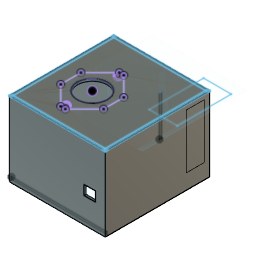
spws box v4 (Autodesk Fusion 360 design; units mm, degrees)
Autodesk Fusion 360 part; units mm, degrees
note: some values were not read from the file. Set by a fixed rule: which sketch regions a step uses.
cylinder "CylinderPrimitive1" add diameter 27.8 height 37 placed x (1, 0, 0) y (0, 1, 0) z (0, 0, 1) at (49.5584, -15.2977, 0) makes body 1
sketch "Sketch2" plane through (0, 0, 0) normal (0, 0, -1) x (1, 0, 0)
  circle A0 centre (49.5584, 15.2977) radius 13.9
  line L0 (38.0977, 16.5) -> (39.0977, 16.5)
  line L1 (39.0977, 16.5) -> (39.0977, 13.5)
  line L2 (39.0977, 13.5) -> (38.0977, 13.5)
  line L3 (38.0977, 13.5) -> (38.0977, 16.5)
  line L4 (60.0977, 16.5) -> (61.0977, 16.5)
  line L5 (61.0977, 16.5) -> (61.0977, 13.5)
  line L6 (61.0977, 13.5) -> (60.0977, 13.5)
  line L7 (60.0977, 13.5) -> (60.0977, 16.5)
  line L8 (35.6613, 15.0104) -> (63.4554, 15.0104) construction
  dimension "d4" = 1
  dimension "d5" = 3
  dimension "d6" = 1
  dimension "d7" = 3
  dimension "d8" = 23
  constraint horizontal L0
  constraint vertical L1
  constraint horizontal L2
  constraint vertical L3
  constraint horizontal L4
  constraint vertical L5
  constraint horizontal L6
  constraint vertical L7
  constraint coincident A0 L8.start
  constraint coincident A0 L8.end
  constraint perpendicular L3 L8
  constraint collinear L0 L4
  measures "d4" distance of L0.start L0.end
  measures "d5" distance of L0.start L2.end
  measures "d6" distance of L4.start L4.end
  measures "d7" distance of L4.start L6.end
  measures "d8" distance of L3 L5
extrude "Extrude1" add sketch "Sketch2" along normal blind 9 contours L0 L1 L2 L3 | L4 L5 L6 L7 bodies 1
sketch "Sketch3" plane through (0, 0, 37) normal (0, 0, 1) x (-1, 0, 0)
  circle A0 centre (-49.5584, 15.2977) radius 13.9
  line L0 (-29.4469, 24.7508) -> (-29.4469, 5.8367)
  line L1 (-29.4469, 5.8367) -> (-47.4256, -12.142)
  line L2 (-51.6682, -12.142) -> (-69.6469, 5.8367)
  line L3 (-69.6469, 5.8367) -> (-69.6469, 24.7508)
  line L4 (-69.6469, 24.7508) -> (-51.6682, 42.7295)
  line L5 (-47.4256, 42.7295) -> (-29.4469, 24.7508)
  line L6 (-49.5469, -14.2633) -> (-49.5469, 44.8508) construction
  line L7 (-29.4469, 15.2937) -> (-69.6469, 15.2937) construction
  arc A1 (-51.6682, -12.142) -> (-47.4256, -12.142) centre (-49.5469, -10.0207) ccw
  arc A2 (-47.4256, 42.7295) -> (-51.6682, 42.7295) centre (-49.5469, 40.6081) ccw
  circle A3 centre (-49.5584, 15.2977) radius 1.15
  circle A4 centre (-49.5469, 39.4977) radius 1.4
  circle A5 centre (-49.5469, -8.9023) radius 1.4
  dimension "d11" = 40.2
  dimension "d14" = 41.8
  dimension "d15" = 41.8
  dimension "d19" = 3
  dimension "d22" = 2.3
  dimension "d29" = 2.8
  dimension "d30" = 2.8
  dimension "d31" = 48.4
  dimension "d32" = 24.2
  constraint perpendicular L1 L2
  constraint parallel L0 L3
  constraint parallel L1 L4
  constraint parallel L2 L5
  constraint vertical L6
  constraint vertical L0
  constraint equal L0 L3
  constraint midpoint L0 L7.start
  constraint midpoint L3 L7.end
  constraint coincident L6.start L2
  constraint coincident L6.start L1
  constraint tangent L2 A1
  constraint tangent L1 A1
  constraint coincident L6.end L4
  constraint coincident L6.end L5
  constraint tangent L4 A2
  constraint tangent L5 A2
  constraint equal A1 A2
  constraint concentric A0 A3
  constraint coincident L6 A4.centre
  constraint coincident L6 A5.centre
  measures "d11" distance of L0 L3
  measures "d14" distance of L1 L4
  measures "d15" distance of L2 L5
  measures "d19" radius of A1
  measures "d22" diameter of A3
  measures "d29" diameter of A4
  measures "d30" diameter of A5
  measures "d31" distance of A4.centre A5.centre
  measures "d32" vertical distance of A0.centre A4.centre
extrude "Extrude2" add sketch "Sketch3" along normal blind 3.2 separate body contours A0 | L0 L1 L2 L3 L4 L5 A1 A2 | A3 makes body 2
extrude "Extrude5" add sketch "Sketch3" along normal blind 23 contours A3 bodies 1 2
sketch "Sketch1" plane through (0, 0, 37) normal (0, 0, 1) x (-1, 0, 0) in component "box"
  line L0 (-104.413, -40) -> (-14.413, -40)
  line L1 (-14.413, -40) -> (-14.413, 58)
  line L2 (-14.413, 58) -> (-104.413, 58)
  line L3 (-104.413, 58) -> (-104.413, -40)
  line L4 (-47.4256, 42.7295) -> (-29.4469, 24.7508)
  line L5 (-29.4469, 24.7508) -> (-29.4469, 5.8367)
  line L6 (-29.4469, 5.8367) -> (-47.4256, -12.142)
  arc A0 (-51.6682, -12.142) -> (-47.4256, -12.142) centre (-49.5469, -10.0207) ccw
  line L7 (-51.6682, -12.142) -> (-69.6469, 5.8367)
  line L8 (-69.6469, 5.8367) -> (-69.6469, 24.7508)
  line L9 (-69.6469, 24.7508) -> (-51.6682, 42.7295)
  arc A1 (-47.4256, 42.7295) -> (-51.6682, 42.7295) centre (-49.5469, 40.6081) ccw
  circle A2 centre (-49.5469, -8.9023) radius 1.4
  circle A3 centre (-49.5469, 39.4977) radius 1.4
  circle A4 centre (-49.5584, 15.2977) radius 13.9
  circle A5 centre (-49.5584, 15.2977) radius 1.15
  circle A6 centre (-49.5584, 15.2977) radius 14.1
  line L10 (-104.413, 58) -> (-14.413, 58)
  line L11 (-14.413, 58) -> (-14.413, 56)
  line L12 (-14.413, 56) -> (-104.413, 56)
  line L13 (-104.413, 56) -> (-104.413, 58)
  line L14 (-104.413, -40) -> (-102.413, -40)
  line L15 (-102.413, -40) -> (-102.413, 58)
  line L16 (-102.413, 58) -> (-104.413, 58)
  line L17 (-104.413, 58) -> (-104.413, -40)
  line L18 (-104.413, -40) -> (-14.413, -40)
  line L19 (-14.413, -40) -> (-14.413, -38)
  line L20 (-14.413, -38) -> (-104.413, -38)
  line L21 (-104.413, -38) -> (-104.413, -40)
  line L22 (-14.413, -40) -> (-16.413, -40)
  line L23 (-16.413, -40) -> (-16.413, 58)
  line L24 (-16.413, 58) -> (-14.413, 58)
  line L25 (-14.413, 58) -> (-14.413, -40)
  dimension "d37" = 2.3
  dimension "d38" = 0.2
  dimension "d43" = 2
  dimension "d46" = 2
  dimension "d53" = 2
  dimension "d56" = 98
  dimension "d57" = 2
  dimension "d86" = 90
  constraint horizontal L0
  constraint vertical L1
  constraint horizontal L2
  constraint vertical L3
  constraint concentric A4 A5
  constraint horizontal L10
  constraint vertical L11
  constraint horizontal L12
  constraint vertical L13
  constraint coincident L1 L11.end
  constraint horizontal L14
  constraint vertical L15
  constraint horizontal L16
  constraint vertical L17
  constraint coincident L10 L15.end
  constraint horizontal L18
  constraint vertical L19
  constraint horizontal L20
  constraint vertical L21
  constraint horizontal L22
  constraint vertical L23
  constraint horizontal L24
  constraint vertical L25
  constraint coincident L10 L23.end
  measures "d37" diameter of A5
  measures "d43" distance of L2.end L12.end
  measures "d46" distance of L3 L15
  measures "d53" distance of L0.start L20.end
  measures "d56" distance of L0.end L1.end
  measures "d57" distance of L23 L25
  measures "d86" distance of L1 L17
extrude "Extrude2'" add sketch "Sketch1" against normal blind 2 separate body contours L0 L3 L14 L15 L17 L18 L20 L21 | L0 L15 L18 L20 L23 | L3 L12 L15 L17 L20 | L0 L1 L18 L19 L20 L22 L23 L25 | L12 L15 L20 L23 | L2 L3 L10 L12 L13 L15 L16 L17 | L1 L12 L20 L23 L25 | L2 L10 L12 L15 L23 | L1 L2 L10 L11 L12 L23 L24 L25 | L4 L5 L6 A0 L7 L8 L9 A1 makes body 3 in component "box"
sketch "Sketch1 (2)" plane through (0, 0, 35) normal (0, 0, -1) x (1, 0, 0) in component "relay"
  circle A0 centre (49.5469, 39.4977) radius 1.4
  circle A1 centre (49.5469, -8.9023) radius 1.4
  circle A2 centre (49.5584, 15.2977) radius 14.1
  line L0 (104.413, -40) -> (104.413, 58)
  line L1 (104.413, 58) -> (14.413, 58)
  line L2 (14.413, 58) -> (14.413, -40)
  line L3 (14.413, -40) -> (104.413, -40)
  line L4 (100, -30) -> (74, -30)
  line L5 (74, -30) -> (74, 21)
  line L6 (74, 21) -> (100, 21)
  line L7 (100, 21) -> (100, -30)
  dimension "d39" = 26
  dimension "d40" = 51
  constraint horizontal L4
  constraint vertical L5
  constraint horizontal L6
  constraint vertical L7
  measures "d39" distance of L4.start L4.end
  measures "d40" distance of L4.start L6.end
extrude "Extrude1'" add sketch "Sketch1 (2)" along normal blind 17 separate body contours L4 L5 L6 L7 makes body 4 in component "relay"
extrude "Extrude3" add sketch "Sketch1" against normal blind 90 separate body contours L2 L3 L10 L12 L13 L15 L16 L17 | L2 L10 L12 L15 L23 | L1 L2 L10 L11 L12 L23 L24 L25 makes body 5 in component "box"
extrude "Extrude4" add sketch "Sketch1" against normal blind 90 contours L0 L3 L14 L15 L17 L18 L20 L21 | L3 L12 L15 L17 L20 | L2 L3 L10 L12 L13 L15 L16 L17 bodies 3 5 in component "box"
sketch "Sketch1 (3)" plane through (102.413, 0, 0) normal (-1, 0, 0) x (0, -1, 0) in component "board"
  line L0 (56, 35) -> (-40, 35)
  line L1 (-40, 35) -> (-40, -53)
  line L2 (-40, -53) -> (56, -53)
  line L3 (56, -53) -> (56, 35)
  line L4 (45.681, 13.1141) -> (-25.319, 13.1141)
  line L5 (-25.319, 13.1141) -> (-25.319, -37.8859)
  line L6 (-25.319, -37.8859) -> (45.681, -37.8859)
  line L7 (45.681, -37.8859) -> (45.681, 13.1141)
  dimension "d49" = 71
  dimension "d50" = 51
  constraint horizontal L4
  constraint vertical L5
  constraint horizontal L6
  constraint vertical L7
  measures "d49" distance of L4.start L4.end
  measures "d50" distance of L4.start L6.end
extrude "Extrude1''" add sketch "Sketch1 (3)" along normal blind 25 separate body contours L4 L5 L6 L7 makes body 6 in component "board"
extrude "Extrude5'" add sketch "Sketch1" against normal blind 70 separate body contours L0 L15 L18 L20 L23 | L0 L1 L18 L19 L20 L22 L23 L25 makes body 7 in component "box"
extrude "Extrude6" add sketch "Sketch1" against normal blind 67 separate body contours L1 L12 L20 L23 L25 makes body 8 in component "box"
move_face "MoveFace1" by (0, -0.1506, 24.0961) 1 faces at (77.413, 1.6524, -3.8859) on bodies 6 in component "board"
move_body "Move1" bodies 4 to x (1, 0, 0) y (0, 0, 1) z (0, -1, 0) at (0, 22.5, 13.5) in component "relay"
move_face "OffsetFaces1" offset -20 1 faces at (103.7464, -24.6667, -53) on bodies 3 in component "box"
sketch "Sketch2 (2)" plane through (0, -58, 0) normal (0, -1, 0) x (1, 0, 0) in component "box"
  line L0 (104.413, 37) -> (14.413, 37)
  line L1 (14.413, 37) -> (14.413, -33)
  line L2 (14.413, -33) -> (104.413, -33)
  line L3 (104.413, -33) -> (104.413, 37)
sketch "Sketch2 (3)" plane through (0, -45.681, 0) normal (0, -1, 0) x (1, 0, 0) in component "board"
  line L0 (102.413, -37.8859) -> (102.413, 13.1141)
  line L1 (102.413, 13.1141) -> (77.413, 13.1141)
  line L2 (77.413, 13.1141) -> (77.413, -37.8859)
  line L3 (77.413, -37.8859) -> (102.413, -37.8859)
  line L4 (84.613, -30.6859) -> (102.413, -30.6859)
  line L5 (102.413, -30.6859) -> (102.413, -21.6859)
  line L6 (102.413, -21.6859) -> (84.613, -21.6859)
  line L7 (84.613, -21.6859) -> (84.613, -30.6859)
  line L8 (95.413, -21.6859) -> (95.413, -30.6859)
  dimension "d61" = 16.2
  dimension "d62" = 9
  dimension "d63" = 17.8
  dimension "d66" = 10.8
  constraint horizontal L4
  constraint vertical L5
  constraint horizontal L6
  constraint vertical L7
  constraint coincident L0 L5.end
  constraint coincident L6 L8.start
  constraint coincident L4 L8.end
  constraint perpendicular L4 L8
  measures "d61" distance of L3 L6
  measures "d62" distance of L4.start L6.end
  measures "d63" distance of L5.end L6.end
  measures "d66" distance of L7 L8
extrude "Extrude7" cut sketch "Sketch2 (3)" along normal blind 4 contours L4 L6 L7 L8 sketch seen with x (1, 0, 0) y (0, 1, 0) z (0, 0, 1) at (-0.2064, -9.9624, 21.576) bodies 3 in component "box"
sketch "Sketch1 (4)" plane through (0, 38, 0) normal (0, -1, 0) x (1, 0, 0) in component "Display"
  line L0 (102.413, 37) -> (14.413, 37)
  line L1 (14.413, 37) -> (14.413, -33)
  line L2 (14.413, -33) -> (102.413, -33)
  line L3 (102.413, -33) -> (102.413, 37)
  line L4 (53.6, -18.3826) -> (65, -18.3826)
  line L5 (65, -18.3826) -> (65, 20.0174)
  line L6 (65, 20.0174) -> (53.6, 20.0174)
  line L7 (53.6, 20.0174) -> (53.6, -18.3826)
  line L8 (53.6, -12.4826) -> (65, -12.4826)
  line L9 (65, -12.4826) -> (65, 14.1174)
  line L10 (65, 14.1174) -> (53.6, 14.1174)
  line L11 (53.6, 14.1174) -> (53.6, -12.4826)
  line L12 (65, -18.3826) -> (67, -18.3826)
  line L13 (67, -18.3826) -> (67, 35)
  line L14 (67, 35) -> (65, 35)
  line L15 (65, 35) -> (65, -18.3826)
  line L16 (14.413, -30) -> (103.413, -30)
  line L17 (103.413, -30) -> (103.413, -32)
  line L18 (103.413, -32) -> (14.413, -32)
  line L19 (14.413, -32) -> (14.413, -30)
  dimension "d67" = 11.4
  dimension "d68" = 38.4
  dimension "d69" = 26.6
  dimension "d70" = 5.9
  dimension "d78" = 2
  dimension "d83" = 1
  dimension "d88" = 89
  constraint horizontal L4
  constraint vertical L5
  constraint horizontal L6
  constraint vertical L7
  constraint horizontal L8
  constraint vertical L9
  constraint horizontal L10
  constraint vertical L11
  constraint coincident L5 L9.end
  constraint coincident L7 L8.start
  constraint horizontal L12
  constraint vertical L13
  constraint horizontal L14
  constraint vertical L15
  constraint horizontal L16
  constraint vertical L17
  constraint horizontal L18
  constraint vertical L19
  constraint coincident L1 L16.start
  measures "d67" distance of L4.start L4.end
  measures "d68" distance of L4.start L6.end
  measures "d69" distance of L8 L10
  measures "d70" distance of L6 L10
  measures "d78" distance of L16.start L18.end
  measures "d83" distance of L2 L18
  measures "d88" distance of L17 L19
extrude "Extrude8" cut sketch "Sketch1 (4)" against normal blind 5 contours L5 L7 L8 L9 L10 L11 L15 bodies 7 in component "box"
extrude "Extrude9" add sketch "Sketch1 (4)" along normal blind 5.8 contours L5 L9 L12 L13 L14 L15 bodies 3 8 7 in component "box"
sketch "Sketch3 (2)" plane through (65, 0, 0) normal (-1, 0, 0) x (0, -1, 0) in component "box"
  line L0 (-40, 14.1174) -> (-40, -12.4826)
  line L1 (-40, -12.4826) -> (-38, -12.4826)
  line L2 (-38, -12.4826) -> (-38, -18.3826)
  line L3 (-38, -18.3826) -> (-32.2, -18.3826)
  line L4 (-32.2, -18.3826) -> (-32.2, 35)
  line L5 (-32.2, 35) -> (-38, 35)
  line L6 (-38, 35) -> (-38, 14.1174)
  line L7 (-38, 14.1174) -> (-40, 14.1174)
  line L8 (-32.2, -18.3826) -> (-34.2, -18.3826)
  line L9 (-34.2, -18.3826) -> (-34.2, 19.8284)
  line L10 (-34.2, 19.8284) -> (-32.2, 19.8284)
  line L11 (-32.2, 19.8284) -> (-32.2, -18.3826)
  dimension "d75" = 2
  constraint horizontal L8
  constraint vertical L9
  constraint horizontal L10
  constraint vertical L11
  constraint coincident L3.end L4.start
  measures "d75" distance of L9 L11
extrude "Extrude10" add sketch "Sketch3 (2)" along normal blind 13 contours L3 L4 L8 L9 L10 L11 bodies 3 in component "box"
extrude "Extrude11" cut sketch "Sketch1 (4)" against normal blind 1 contours L3 L16 L17 L18 | L1 L3 L16 L18 L19 bodies 3 in component "box"
sketch "Sketch4" plane through (0, -56, 0) normal (0, 1, 0) x (-1, 0, 0) in component "box"
  line L0 (-95.2067, -0.1098) -> (-84.4067, -0.1098)
  line L1 (-84.4067, -0.1098) -> (-84.4067, -9.1098)
  line L2 (-84.4067, -9.1098) -> (-95.2067, -9.1098)
  line L3 (-95.2067, -9.1098) -> (-95.2067, -0.1098)
  line L4 (-102.413, 35) -> (-102.413, -33)
  line L5 (-102.413, -33) -> (-14.413, -33)
  line L6 (-14.413, -33) -> (-14.413, 35)
  line L7 (-14.413, 35) -> (-102.413, 35)
  line L8 (-14.413, -30) -> (-103.413, -30)
  line L9 (-103.413, -30) -> (-103.413, -32)
  line L10 (-103.413, -32) -> (-14.413, -32)
  line L11 (-14.413, -32) -> (-14.413, -30)
  dimension "d81" = 2
  dimension "d82" = 3
  dimension "d87" = 89
  constraint horizontal L8
  constraint vertical L9
  constraint horizontal L10
  constraint vertical L11
  constraint coincident L6 L8.start
  measures "d81" distance of L8.start L10.end
  measures "d82" distance of L5 L8
  measures "d87" distance of L9 L11
sketch "Sketch5" plane through (102.413, 0, 0) normal (-1, 0, 0) x (0, -1, 0) in component "box"
  line L0 (-38, 35) -> (-38, -30)
  line L1 (-38, -30) -> (-38, -32)
  line L2 (-38, -32) -> (-38, -33)
  line L3 (-38, -33) -> (56, -33)
  line L4 (56, -33) -> (56, 35)
  line L5 (56, 35) -> (-38, 35)
  line L6 (-38, -30) -> (56, -30)
  line L7 (56, -30) -> (56, -32)
  line L8 (56, -32) -> (-38, -32)
  line L9 (-38, -32) -> (-38, -30)
  dimension "d89" = 2
  constraint horizontal L6
  constraint vertical L7
  constraint horizontal L8
  constraint vertical L9
  constraint coincident L4 L7.end
  constraint coincident L0.end L1.start
  measures "d89" distance of L6 L8
extrude "Extrude13" cut sketch "Sketch5" against normal blind 1 contours L1 L4 L6 L7 L8 L9 bodies 3 in component "box"
extrude "Extrude14" cut sketch "Sketch4" against normal blind 1 contours L4 L6 L8 L10 L11 bodies 3 in component "box"
sketch "Sketch1 (5)" plane through (0, 0, -30) normal (0, 0, -1) x (1, 0, 0) in component "BACK WALL"
  line L0 (14.413, 56) -> (14.413, -38)
  line L1 (14.413, -38) -> (16.413, -38)
  line L2 (16.413, -38) -> (16.413, 56)
  line L3 (16.413, 56) -> (14.413, 56)
  line L4 (14.7, -38.9988) -> (103.5, -38.9988)
  line L5 (103.5, -38.9988) -> (103.5, 56.6012)
  line L6 (103.5, 56.6012) -> (14.7, 56.6012)
  line L7 (14.7, 56.6012) -> (14.7, -38.9988)
  dimension "d94" = 95.6
  dimension "d95" = 88.8
  constraint horizontal L4
  constraint vertical L5
  constraint horizontal L6
  constraint vertical L7
  measures "d94" distance of L4 L6
  measures "d95" distance of L5 L7
extrude "Extrude1'''" add sketch "Sketch1 (5)" along normal blind 1.8 separate body contours L1 L2 L3 L4 L5 L6 L7 | L1 L2 L3 L7 makes body 9 in component "BACK WALL"
extrude "Extrude12" cut sketch "Sketch4" against normal blind 1 contours L4 L6 L8 L10 L11 bodies 3 in component "box"
combine "Combine1" operation add target body 8 tool bodies 3 in component "box"
sketch "Sketch4 (2)" plane through (0, 0, 0) normal (1, 0, 0) x (0, 1, 0)
component "box" placed x (1, 0, 0) y (0, 1, 0) z (0, 0, 1) at (0, 0, 0)
component "relay" placed x (1, 0, 0) y (0, 1, 0) z (0, 0, 1) at (3.921, 30.7276, -11.4012)
component "board" placed x (1, 0, 0) y (0, 1, 0) z (0, 0, 1) at (-0.2064, -9.9624, 21.576)
component "Display" placed x (1, 0, 0) y (0, 1, 0) z (0, 0, 1) at (0, 0, 0)
component "BACK WALL" placed x (1, 0, 0) y (0, 1, 0) z (0, 0, 1) at (0, 0, 0)
equation "d63 = 10.8 mm + 7 mm"
